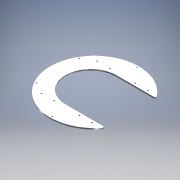
# Autodesk Inventor part: Turret Support
Saved by Autodesk Inventor 2019.4 (Build 234330000, 330)
## iProperties
Created: 2020-01-19
Part Number: Turret Support
Material: Aluminum 6061
Document SubType Name: Modeling
Designer: Mark
Mass: 597.772 g
Surface Area: 967.523 cm^2
Volume: 221.397 cm^3
Density: 2.7 g/cm^3
Appearance: Aluminum - Flat
Author: Mark
Autodesk Inventor part; units mm, degrees
ref_plane "YZ Plane" through (0, 0, 0) normal (1, 0, 0) x (0, 1, 0)
ref_plane "XZ Plane" through (0, 0, 0) normal (0, 1, 0) x (-1, 0, 0)
ref_plane "XY Plane" through (0, 0, 0) normal (0, 0, 1) x (1, 0, 0)
sketch "Sketch1" plane through (0, 0, 0) normal (0, 1, 0) x (-1, 0, 0)
  circle A0 centre (0, 0) radius 175
  dimension "d0" = 350
  constraints: 1 centre point, 1 coincident
  measures "d0" diameter of A0
extrude "Extrusion1" add sketch "Sketch1" along normal blind 5
sketch "Sketch2" plane through (0, 5, 0) normal (0, 1, 0) x (1, 0, 0)
  line L0 (-50, 110) -> (50, 110)
  line L1 (50, 110) -> (50, -110)
  line L2 (50, -110) -> (-50, -110)
  line L3 (-50, -110) -> (-50, 110)
  line L4 (-50, 110) -> (50, -110) construction
  line L5 (50, 110) -> (-50, -110) construction
  line L6 (-100, 110) -> (100, 110)
  line L7 (100, 110) -> (100, -110)
  line L8 (100, -110) -> (-100, -110)
  line L9 (-100, -110) -> (-100, 110)
  line L10 (-100, 110) -> (100, -110) construction
  line L11 (100, 110) -> (-100, -110) construction
  circle A0 centre (-100, 110) radius 2.75
  circle A1 centre (-50, 110) radius 2.75
  circle A2 centre (50, 110) radius 2.75
  circle A3 centre (100, 110) radius 2.75
  circle A4 centre (100, -110) radius 2.75
  circle A5 centre (50, -110) radius 2.75
  circle A6 centre (-50, -110) radius 2.75
  circle A7 centre (-100, -110) radius 2.75
  point P0 (0, 0)
  dimension "d3" = 220
  dimension "d4" = 100
  dimension "d5" = 200
  dimension "d6" = 220
  dimension "d7" = 5.5
  dimension "d8" = 5.5
  dimension "d9" = 5.5
  dimension "d10" = 5.5
  dimension "d11" = 5.5
  dimension "d12" = 5.5
  dimension "d13" = 5.5
  dimension "d14" = 5.5
  constraints: 24 end point, 8 centre point, 8 coincident, 4 midpoint, 4 parallel, 2 horizontal, 2 perpendicular
  measures "d3" distance of L0.end L1.end
  measures "d4" distance of L1.end L2.end
  measures "d5" distance of L7.end L8.end
  measures "d6" distance of L8.end L6.start
  measures "d7" diameter of A0
  measures "d8" diameter of A1
  measures "d9" diameter of A2
  measures "d10" diameter of A3
  measures "d11" diameter of A4
  measures "d12" diameter of A5
  measures "d13" diameter of A6
  measures "d14" diameter of A7
extrude "Extrusion2" cut sketch "Sketch2" against normal blind 5 contours L6 A1 L0 | L0 A1 L3 | L3 A1 L6 | A2 L6 L0 | L0 L1 A2 | A6 L2 L3 | L3 L8 A6 | A0 L9 L6 | L6 L9 A0 | L6 A2 L1 | L2 A6 L8 | A3 L7 L6 | L6 L7 A3 | A5 L8 L1 | L1 L2 A5 | L2 L8 A5 | A7 L9 L8 | L8 L9 A7 | A4 L8 L7 | L7 L8 A4
sketch "Sketch3" plane through (0, 5, 0) normal (0, 1, 0) x (1, 0, 0)
  line L0 (-115, 100) -> (115, 100)
  line L1 (115, 100) -> (115, -100)
  line L2 (115, -100) -> (-115, -100)
  line L3 (-115, -100) -> (-115, 100)
  line L4 (-115, 100) -> (115, -100) construction
  line L5 (115, 100) -> (-115, -100) construction
  line L6 (115, 100) -> (235, 100)
  line L7 (235, 100) -> (235, -100)
  line L8 (235, -100) -> (115, -100)
  line L9 (115, -100) -> (115, 100)
  point P0 (0, 0)
  dimension "d17" = 230
  dimension "d18" = 200
  dimension "d19" = 120
  dimension "d20" = 200
  constraints: 20 end point, 4 parallel, 2 horizontal, 2 midpoint, 2 perpendicular
  measures "d17" distance of L1.end L2.end
  measures "d18" distance of L0.end L1.end
  measures "d19" distance of L7.end L8.end
  measures "d20" distance of L6.end L7.end
extrude "Extrusion3" cut sketch "Sketch3" against normal blind 5
fillet "Fillet1" radius 100 2 edges at (-115, 2.5, 100) (-115, 2.5, -100)
fillet "Fillet2" radius 5 2 edges at (143.6141, 2.5, 100) (143.6141, 2.5, -100)
sketch "Sketch4" plane through (0, 5, 0) normal (0, 1, 0) x (1, 0, 0)
  circle A0 centre (0, 0) radius 168.25 construction
  circle A1 centre (0, 168.25) radius 2.75
  line L0 (0, 0) -> (0, 168.25) construction
  line L1 (0, 0) -> (168.25, 0) construction
  circle A2 centre (-145.7088, 84.125) radius 2.75
  circle A3 centre (-145.7088, -84.125) radius 2.75
  circle A4 centre (0, -168.25) radius 2.75
  circle A5 centre (145.7088, -84.125) radius 2.75
  circle A6 centre (145.7088, 84.125) radius 2.75
  dimension "d25" = 336.5
  dimension "d26" = 5.5
  dimension "d27" = 90
  dimension "d30" = 360
  constraints: 6 centre point, 4 end point, 1 coincident, 1 horizontal, 1 perpendicular, 1 vertical alignment, 15 other
  measures "d26" diameter of A1
  measures "d27" angle of L1 L0
extrude "Extrusion4" cut sketch "Sketch4" against normal blind 10 contours A1 | A2 | A3 | A4 | A6
body "Solid1"
